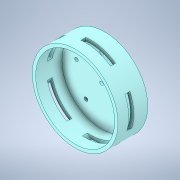
# Autodesk Inventor part: Wheel1
Saved by Autodesk Inventor 2020.1 (Build 241239000, 239)
## iProperties
Created: 2019-11-14
Part Number: Wheel1
Material: Generic
Document SubType Name: Modeling
Designer: Ali
Density: 1 g/cm^3
Appearance: Default
Author: Ali
Autodesk Inventor part; units mm, degrees
ref_plane "YZ Plane" through (0, 0, 0) normal (1, 0, 0) x (0, 1, 0)
ref_plane "XZ Plane" through (0, 0, 0) normal (0, 1, 0) x (-1, 0, 0)
sketch "Sketch1" plane through (0, 0, 0) normal (0, 0, 1) x (1, 0, 0)
  line L0 (0, 0) -> (50.8, 0) construction
  line L1 (0, 82.55) -> (0, 76.2)
  line L2 (0, 76.2) -> (50.8, 76.2)
  line L3 (50.8, 76.2) -> (50.8, 82.55)
  line L4 (50.8, 82.55) -> (0, 82.55)
  dimension "d1" = 50.8
  dimension "d7" = 76.2
  dimension "d8" = 6.35
  constraints: 10 end point, 2 perpendicular, 2 vertical, 1 horizontal
  measures "d1" distance of L1.end L2.end
  measures "d7" distance between parallel lines of L0 L2
  measures "d8" distance of L1.start L1.end
revolve "Revolution1" add sketch "Sketch1" angle 360 about axis through (0, 0, 0) along (1, 0, 0)
sketch "Sketch2" plane through (50.8, 0, 0) normal (1, 0, 0) x (0, 0, -1)
  circle A0 centre (0, 0) radius 82.55 projected
  circle A1 centre (0, 0) radius 76.2 projected
extrude "Extrusion1" add sketch "Sketch2" along normal blind 6.35 contours A0 | A1
sketch "Sketch3" plane through (50.8, 0, 0) normal (-1, 0, 0) x (0, 0, 1)
  point P0 (0, 0)
  point P1 (0, 50.8)
  point P2 (0, 0)
  dimension "d9" = 50.8
  constraints: 1 coincident
  measures "d9" distance of point (0, 0) point (0, 50.8)
hole "Hole1" at (50.8, 50.8, 0) at (50.8, 0, 0) direction (1, 0, 0) diameter 6.858 end through all
pattern_circular "Circular Pattern1" count 5 over 360 about axis through (25.4, 0, 0) along (1, 0, 0) of "Hole1"
ref_plane "Work Plane1" through (25.4, 0, 0) normal (-1, 0, 0) x (0, 0, 1)
sketch "Sketch5" plane through (25.4, 0, 0) normal (-1, 0, 0) x (0, 0, 1)
  circle A0 centre (0, 0) radius 76.2 projected
  circle A1 centre (0, 0) radius 82.55 projected
  circle A2 centre (48.3137, 15.6981) radius 3.429 projected
  circle A3 centre (29.8595, -41.0981) radius 3.429 projected
  circle A4 centre (0, 50.8) radius 3.429 construction
  circle A5 centre (0, 0) radius 3.429 projected
  circle A6 centre (0, 0) radius 76.2 projected
  circle A7 centre (0, 50.8) radius 3.429 construction
  circle A8 centre (0, 50.8) radius 9.525 construction
  line L0 (0, 60.325) -> (49.1356, 60.325) construction
  line L1 (49.1356, 60.325) -> (49.1356, 41.275) construction
  line L2 (49.1356, 41.275) -> (0, 41.275) construction
  line L3 (0, 41.275) -> (0, 60.325) construction
  circle A9 centre (0, 50.8) radius 50.4056 construction
  circle A10 centre (0, 0) radius 76.2 projected
  arc A11 (49.9526, 57.5428) -> (47.5712, 67.4647) centre (0, 50.8) ccw
  line L4 (-9.525, 50.8) -> (-9.525, 81.9986) construction
  circle A12 centre (0, 0) radius 76.2 projected
  line L5 (-9.525, 75.6023) -> (-9.525, 81.9986)
  arc A13 (49.9526, 57.5428) -> (-9.525, 75.6023) centre (0, 0) ccw
  arc A14 (47.5712, 67.4647) -> (-9.525, 81.9986) centre (0, 0) ccw
  point P0 (49.9526, 57.5428)
  dimension "d27" = 19.05
  dimension "d28" = 19.05
  dimension "d29" = 49.1356
  dimension "d30" = 100.8113
  dimension "d31" = 82.55
  constraints: 13 point on circle, 12 end point, 5 centre point, 2 coincident, 2 concentric, 2 parallel, 2 vertical, 1 horizontal, 1 perpendicular, 1 point on line, 1 tangent, 2 other
  measures "d27" diameter of A8
  measures "d28" distance of L2.end L0.start
  measures "d29" distance of L1.end L2.end
  measures "d30" diameter of A9
  measures "d31" radius of A14
extrude "Extrusion2" cut sketch "Sketch5" along normal mid plane 9.525 contours A0 L5 A1 A11 picked at (-1.9672, 80.2341)
pattern_circular "Circular Pattern2" count 5 over 360 about axis through (291.1792, 0, 0) along (-1, 0, 0) of "Extrusion2"
equation "\"d1\" = wheelDepth"
equation "\"d7\" = wheelR"
equation "\"d8\" = wheelThickness"
equation "\"d9\" = farFromCenter"
equation "\"d10\" = smallHoles"
equation "\"d27\" = swivelBaseDiameter"
equation "\"d28\" = d27"
equation "\"d29\" = swivelLegLength"
equation "\"d31\" = wheelR + wheelThickness"
equation "\"d32\" = 0.5 * swivelLegThickness"
equation "\"gearShaft\" = 6.35"
equation "\"largeGear\" = 38.1"
equation "\"smallGear\" = 12.7"
equation "\"wheelR\" = 76.2"
equation "\"wheelThickness\" = 6.35"
equation "\"wheelDepth\" = 50.8"
equation "\"mainHole\" = 6.858"
equation "\"smallHoles\" = 6.858"
equation "\"farFromCenter\" = 50.8"
equation "\"smallGearLength\" = 50.8"
equation "\"mainGearLength\" = 76.2"
equation "\"gearThickness\" = 6.35"
equation "\"mainGear\" = 38.1"
equation "\"d20\" = -0.5 * wheelDepth"
equation "\"swivelBaseDiameter\" = 19.05"
equation "\"swivelLegExtentions\" = 19.05"
equation "\"swivelLegLength\" = 49.13565"
equation "\"swivelLegThickness\" = 19.05"
body "Solid1"
